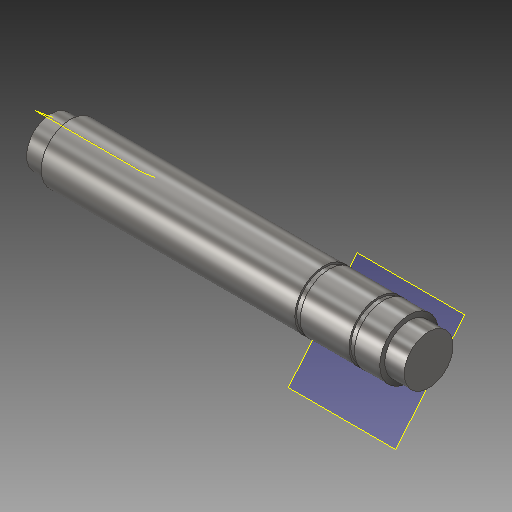
# Autodesk Inventor part: Bevel - Spur Axle
Saved by Autodesk Inventor 2019.4 (Build 234330000, 330)
## iProperties
Created: 2019-11-30
Part Number: Bevel - Spur Axle
Material: Steel, Mild
Document SubType Name: Modeling
Designer: admin
Density: 7.85 g/cm^3
Appearance: Semi-Polished
Mass: 66.5466 g
Surface Area: 30.9384 cm^2
Volume: 8.47727 cm^3
Author: admin
Autodesk Inventor part; units mm, degrees
ref_plane "YZ Plane" through (0, 0, 0) normal (1, 0, 0) x (0, 1, 0)
ref_plane "XZ Plane" through (0, 0, 0) normal (0, 1, 0) x (-1, 0, 0)
ref_plane "XY Plane" through (0, 0, 0) normal (0, 0, 1) x (1, 0, 0)
sketch "Sketch1" plane through (0, 0, 0) normal (0, 0, 1) x (1, 0, 0)
  line L0 (0, 0) -> (0, 5)
  line L1 (0, 5) -> (4, 5)
  line L2 (4, 5) -> (4, 6)
  line L3 (73.4, 6) -> (73.4, 5)
  line L4 (73.4, 5) -> (77.4, 5)
  line L5 (77.4, 5) -> (77.4, 0)
  line L6 (77.4, 0) -> (0, 0)
  line L7 (4, 6) -> (56, 6)
  line L8 (56, 6) -> (56, 5.65)
  line L9 (56, 5.65) -> (57.1, 5.65)
  line L10 (57.1, 5.65) -> (57.1, 6)
  line L11 (57.1, 6) -> (67.1, 6)
  line L12 (67.1, 6) -> (67.1, 5.65)
  line L13 (67.1, 5.65) -> (68.2, 5.65)
  line L14 (68.2, 5.65) -> (68.2, 6)
  line L15 (68.2, 6) -> (73.4, 6)
  dimension "d0" = 5
  dimension "d2" = 69.4
  dimension "d3" = 4
  dimension "d4" = 4
  dimension "d7" = 10
  dimension "d8" = 1.1
  dimension "d9" = 0.35
  dimension "d10" = 1.1
  dimension "d11" = 6
  dimension "d12" = 57.1
  constraints: 32 end point, 10 perpendicular, 7 point on line, 2 horizontal, 1 vertical
  measures "d0" distance between parallel lines of L6 L1
  measures "d2" distance of L2.end L3.start
  measures "d3" distance of L0.end L1.end
  measures "d4" distance of L3.end L4.end
  measures "d7" distance of L10.end L11.end
  measures "d8" distance of L8.end L9.end
  measures "d9" distance of L7.end L8.end
  measures "d10" distance of L12.end L13.end
  measures "d11" distance between parallel lines of L6 L7
  measures "d12" distance between parallel lines of L0 L10
revolve "Revolution1" add sketch "Sketch1" angle 360 about axis through (77.4, 0, 0) along (-1, 0, 0)
ref_plane "Work Plane2" through (11.7403, 0.7528, -4.5479) normal (0, 0.7660444, -0.6427876) x (1, 0, 0)
sketch "Sketch2" plane through (11.7403, 0.7528, -4.5479) normal (0, 0.7660444, -0.6427876) x (1, 0, 0)
  line L0 (0, 0) -> (10, 0) projected
  arc A0 (0, 0) -> (0, -6) centre (0, -3) ccw projected
  line L1 (10, -6) -> (0, -6) projected
  arc A1 (10, -6) -> (10, 0) centre (10, -3) ccw projected
  point P0 (-11.7403, -3)
extrude "Extrusion1" cut sketch "Sketch2" against normal blind 1
ref_plane "Work Plane1" through (65.9621, -4.5479, -0.7528) normal (0, -0.6427876, -0.7660444) x (-1, 0, 0)
sketch "Sketch3" plane through (65.9621, -4.5479, -0.7528) normal (0, -0.6427876, -0.7660444) x (-1, 0, 0)
  line L0 (8, 0) -> (0, 0) projected
  arc A0 (8, 0) -> (8, 6) centre (8, 3) ccw projected
  line L1 (0, 6) -> (8, 6) projected
  arc A1 (0, 6) -> (0, 0) centre (0, 3) ccw projected
  point P0 (65.9621, 3)
extrude "Extrusion2" cut sketch "Sketch3" against normal blind 1
body "Solid1"
